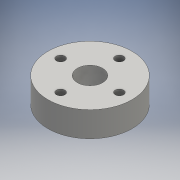
# Autodesk Inventor part: Gear20
Saved by Autodesk Inventor 2016 (Build 200138000, 138)
## iProperties
Created: 2016-11-07
Part Number: Gear20
Material: 一般
Document SubType Name: Modeling
Designer: Daisuke
Density: 1 g/cm^3
Appearance: 既定
Author: Daisuke
Autodesk Inventor part; units mm, degrees
ref_plane "YZ Plane" through (0, 0, 0) normal (1, 0, 0) x (0, 1, 0)
ref_plane "XZ Plane" through (0, 0, 0) normal (0, 1, 0) x (-1, 0, 0)
ref_plane "XY Plane" through (0, 0, 0) normal (0, 0, 1) x (1, 0, 0)
sketch "スケッチ1" plane through (0, 0, 0) normal (0, 0, 1) x (1, 0, 0)
  circle A0 centre (0, 0) radius 3
  circle A1 centre (0, 0) radius 10
  dimension "d0" = 6
  dimension "d1" = 20
  constraints: 2 centre point, 2 coincident
  measures "d0" diameter of A0
  measures "d1" diameter of A1
extrude "押し出し1" add sketch "スケッチ1" along normal blind 6
sketch "スケッチ3" plane through (0, 0, 6) normal (0, 0, 1) x (1, 0, 0)
  circle A0 centre (0, 0) radius 10
  circle A1 centre (0, 0) radius 7 construction
  circle A2 centre (-7, 0) radius 1
  circle A3 centre (-4.9497, -4.9497) radius 1
  circle A4 centre (4.9497, -4.9497) radius 1
  circle A5 centre (0, -7) radius 1
  circle A6 centre (7, 0) radius 1
  circle A7 centre (4.9497, 4.9497) radius 1
  circle A8 centre (0, 7) radius 1
  circle A9 centre (-4.9497, 4.9497) radius 1
  circle A10 centre (0, 0) radius 5
  circle A11 centre (0, 0) radius 10
  circle A12 centre (0, 0) radius 7 construction
  circle A13 centre (-7, 0) radius 1
  circle A14 centre (-4.9497, -4.9497) radius 1
  circle A15 centre (4.9497, -4.9497) radius 1
  circle A16 centre (0, -7) radius 1
  circle A17 centre (7, 0) radius 1
  circle A18 centre (4.9497, 4.9497) radius 1
  circle A19 centre (0, 7) radius 1
  circle A20 centre (-4.9497, 4.9497) radius 1
  circle A21 centre (0, 0) radius 5
  dimension "d9" = 14
  dimension "d20" = 14
  dimension "d8" = 20
  dimension "d10" = 2
  dimension "d11" = 2
  dimension "d12" = 2
  dimension "d13" = 2
  dimension "d14" = 2
  dimension "d15" = 2
  dimension "d16" = 2
  dimension "d17" = 2
  dimension "d18" = 10
  dimension "d19" = 20
  dimension "d21" = 2
  dimension "d22" = 2
  dimension "d23" = 2
  dimension "d24" = 2
  dimension "d25" = 2
  dimension "d26" = 2
  dimension "d27" = 2
  dimension "d28" = 2
  dimension "d29" = 10
  constraints: 20 centre point, 6 coincident, 2 horizontal alignment, 4 other
  measures "d8" diameter of A0
  measures "d10" diameter of A2
  measures "d11" diameter of A3
  measures "d12" diameter of A5
  measures "d13" diameter of A4
  measures "d14" diameter of A6
  measures "d15" diameter of A7
  measures "d16" diameter of A8
  measures "d17" diameter of A9
  measures "d18" diameter of A10
  measures "d19" diameter of A11
  measures "d21" diameter of A13
  measures "d22" diameter of A14
  measures "d23" diameter of A16
  measures "d24" diameter of A15
  measures "d25" diameter of A17
  measures "d26" diameter of A18
  measures "d27" diameter of A19
  measures "d28" diameter of A20
  measures "d29" diameter of A21
extrude "押し出し3" cut sketch "スケッチ3" against normal blind 10 contours A2 | A5 | A6 | A8
